Autodesk Fusion 360 part; units mm, degrees
note: some values were not read from the file. Set by a fixed rule: which sketch regions a step uses.
(part 4 of 4)
  spline S327 degree 3 poles (-0.4705, -4.8236) (-0.4586, -4.7125) (-0.5896, -4.4664) (-0.7999, -4.2085) knots 0 0 0 0 1 1 1 1
  line L146 (-0.7999, -4.2085) -> (-0.9586, -4.018)
  line L147 (-0.9586, -4.018) -> (-1.2563, -4.014)
  spline S328 degree 3 poles (-1.2563, -4.014) (-1.4508, -4.014) (-1.6532, -3.9822) (-1.8437, -3.9267) knots 0 0 0 0 1 1 1 1
  spline S329 degree 3 poles (-1.8437, -3.9267) (-2.1771, -3.8235) (-2.1929, -3.8275) (-2.4509, -4.1053) knots 0 0 0 0 1 1 1 1
  spline S330 degree 3 poles (-2.4509, -4.1053) (-2.7366, -4.4109) (-2.7803, -4.4902) (-2.7525, -4.6927) knots 0 0 0 0 1 1 1 1
  spline S331 degree 3 poles (-2.7525, -4.6927) (-2.7208, -4.9189) (-2.5461, -5.3316) (-2.4191, -5.4824) knots 0 0 0 0 1 1 1 1
  spline S332 degree 3 poles (-2.4191, -5.4824) (-2.3041, -5.6213) (-2.3199, -5.6848) (-2.4707, -5.6848) knots 0 0 0 0 1 1 1 1
  spline S333 degree 3 poles (-2.4707, -5.6848) (-2.57, -5.6848) (-2.5977, -5.6571) (-2.6771, -5.4983) knots 0 0 0 0 1 1 1 1
  spline S334 degree 3 poles (-2.6771, -5.4983) (-2.7366, -5.3634) (-2.7882, -5.3078) (-2.8438, -5.3078) knots 0 0 0 0 1 1 1 1
  spline S335 degree 3 poles (-2.8438, -5.3078) (-2.9351, -5.3078) (-2.9351, -5.2959) (-2.9232, -5.792) knots 0 0 0 0 1 1 1 1
  spline S336 degree 3 poles (-2.9232, -5.792) (-2.9192, -6.0023) (-2.9271, -6.1928) (-2.9391, -6.2167) knots 0 0 0 0 1 1 1 1
  spline S337 degree 3 poles (-2.9391, -6.2167) (-2.9589, -6.2444) (-2.9986, -6.2444) (-3.0621, -6.2127) knots 0 0 0 0 1 1 1 1
  spline S338 degree 3 poles (-3.0621, -6.2127) (-3.1772, -6.1611) (-3.2407, -5.9746) (-3.2407, -5.6967) knots 0 0 0 0 1 1 1 1
  spline S339 degree 3 poles (-3.2407, -5.6967) (-3.2407, -5.5896) (-3.2566, -5.5062) (-3.2724, -5.5062) knots 0 0 0 0 1 1 1 1
  spline S340 degree 3 poles (-3.2724, -5.5062) (-3.3359, -5.5062) (-3.4748, -5.6848) (-3.5502, -5.8674) knots 0 0 0 0 1 1 1 1
  spline S341 degree 3 poles (-3.5502, -5.8674) (-3.6455, -6.0897) (-3.7765, -6.1968) (-3.8836, -6.1373) knots 0 0 0 0 1 1 1 1
  spline S342 degree 3 poles (-3.8836, -6.1373) (-3.9789, -6.0857) (-3.9749, -5.9706) (-3.8598, -5.792) knots 0 0 0 0 1 1 1 1
  spline S343 degree 3 poles (-3.8598, -5.792) (-3.7526, -5.6174) (-3.6891, -5.3872) (-3.7526, -5.3872) knots 0 0 0 0 1 1 1 1
  spline S344 degree 3 poles (-3.7526, -5.3872) (-3.7765, -5.3872) (-3.8519, -5.4507) (-3.9233, -5.534) knots 0 0 0 0 1 1 1 1
  spline S345 degree 3 poles (-3.9233, -5.534) (-4.221, -5.8674) (-4.3162, -5.9428) (-4.4353, -5.9428) knots 0 0 0 0 1 1 1 1
  spline S346 degree 3 poles (-4.4353, -5.9428) (-4.6377, -5.9428) (-4.5901, -5.788) (-4.2805, -5.4388) knots 0 0 0 0 1 1 1 1
  spline S347 degree 3 poles (-4.2805, -5.4388) (-4.1297, -5.2681) (-3.9789, -5.1054) (-3.9431, -5.0737) knots 0 0 0 0 1 1 1 1
  spline S348 degree 3 poles (-3.9431, -5.0737) (-3.9035, -5.0459) (-3.8757, -4.9784) (-3.8757, -4.9308) knots 0 0 0 0 1 1 1 1
  spline S349 degree 3 poles (-3.8757, -4.9308) (-3.8757, -4.8435) (-3.8876, -4.8395) (-4.1257, -4.8435) knots 0 0 0 0 1 1 1 1
  spline S350 degree 3 poles (-4.1257, -4.8435) (-4.4075, -4.8514) (-4.4631, -4.78) (-4.2527, -4.6807) knots 0 0 0 0 1 1 1 1
  spline S351 degree 3 poles (-4.2527, -4.6807) (-4.1892, -4.649) (-4.0821, -4.5974) (-4.0225, -4.5696) knots 0 0 0 0 1 1 1 1
  spline S352 degree 3 poles (-4.0225, -4.5696) (-3.959, -4.5379) (-3.84, -4.5141) (-3.7526, -4.5141) knots 0 0 0 0 1 1 1 1
  spline S353 degree 3 poles (-3.7526, -4.5141) (-3.6256, -4.5141) (-3.5621, -4.4823) (-3.3836, -4.3275) knots 0 0 0 0 1 1 1 1
  spline S354 degree 3 poles (-3.3836, -4.3275) (-3.2566, -4.2164) (-3.1653, -4.1013) (-3.1653, -4.0537) knots 0 0 0 0 1 1 1 1
  spline S355 degree 3 poles (-3.1653, -4.0537) (-3.1573, -3.887) (-2.9232, -3.4901) (-2.7366, -3.3393) knots 0 0 0 0 1 1 1 1
  spline S356 degree 3 poles (-2.7366, -3.3393) (-2.5184, -3.1607) (-2.2604, -3.0853) (-1.8675, -3.0853) knots 0 0 0 0 1 1 1 1
  spline S357 degree 3 poles (-1.8675, -3.0853) (-1.6532, -3.0853) (-1.5619, -3.0694) (-1.4984, -3.0178) knots 0 0 0 0 1 1 1 1
  line L148 (-1.4984, -3.0178) -> (-1.4111, -2.9464)
  line L149 (-1.4111, -2.9464) -> (-1.4944, -2.7083)
  spline S358 degree 3 poles (-1.4944, -2.7083) (-1.6413, -2.2955) (-1.7008, -1.9026) (-1.6968, -1.3589) knots 0 0 0 0 1 1 1 1
  spline S359 degree 3 poles (-1.6968, -1.3589) (-1.6968, -0.7477) (-1.5936, -0.2715) (-1.3436, 0.2603) knots 0 0 0 0 1 1 1 1
  line L150 (-1.3436, 0.2603) -> (-1.1888, 0.5937)
  line L151 (-1.1888, 0.5937) -> (-1.3516, 0.558)
  spline S360 degree 3 poles (-1.3516, 0.558) (-1.4389, 0.5342) (-1.6611, 0.5263) (-1.8437, 0.5382) knots 0 0 0 0 1 1 1 1
  spline S361 degree 3 poles (-1.8437, 0.5382) (-2.2644, 0.562) (-2.5858, 0.7048) (-2.6692, 0.9073) knots 0 0 0 0 1 1 1 1
  spline S362 degree 3 poles (-2.6692, 0.9073) (-2.7446, 1.0819) (-2.7406, 1.5462) (-2.6612, 2.0542) knots 0 0 0 0 1 1 1 1
  spline S363 degree 3 poles (-2.6612, 2.0542) (-2.5938, 2.4948) (-2.6017, 2.59) (-2.7128, 2.59) knots 0 0 0 0 1 1 1 1
  spline S364 degree 3 poles (-2.7128, 2.59) (-2.8795, 2.59) (-3.0383, 2.4352) (-3.1811, 2.1376) knots 0 0 0 0 1 1 1 1
  spline S365 degree 3 poles (-3.1811, 2.1376) (-3.328, 1.828) (-3.4193, 1.7407) (-3.5701, 1.7645) knots 0 0 0 0 1 1 1 1
  spline S366 degree 3 poles (-3.5701, 1.7645) (-3.709, 1.7843) (-3.705, 1.955) (-3.5582, 2.0939) knots 0 0 0 0 1 1 1 1
  spline S367 degree 3 poles (-3.5582, 2.0939) (-3.4272, 2.2169) (-3.3994, 2.3519) (-3.5066, 2.3519) knots 0 0 0 0 1 1 1 1
  spline S368 degree 3 poles (-3.5066, 2.3519) (-3.5423, 2.3519) (-3.6852, 2.3082) (-3.8201, 2.2527) knots 0 0 0 0 1 1 1 1
  spline S369 degree 3 poles (-3.8201, 2.2527) (-4.0543, 2.1574) (-4.3638, 2.1138) (-4.4154, 2.1653) knots 0 0 0 0 1 1 1 1
  spline S370 degree 3 poles (-4.4154, 2.1653) (-4.4829, 2.2288) (-4.3757, 2.3519) (-4.221, 2.3916) knots 0 0 0 0 1 1 1 1
  spline S371 degree 3 poles (-4.221, 2.3916) (-3.9947, 2.4471) (-3.6931, 2.6019) (-3.7169, 2.6495) knots 0 0 0 0 1 1 1 1
  spline S372 degree 3 poles (-3.7169, 2.6495) (-3.7288, 2.6694) (-3.7646, 2.6853) (-3.7963, 2.6773) knots 0 0 0 0 1 1 1 1
  spline S373 degree 3 poles (-3.7963, 2.6773) (-4.0582, 2.6218) (-4.3083, 2.594) (-4.6416, 2.594) knots 0 0 0 0 1 1 1 1
  spline S374 degree 3 poles (-4.6416, 2.594) (-5.0187, 2.59) (-5.0306, 2.594) (-5.0187, 2.6773) knots 0 0 0 0 1 1 1 1
  spline S375 degree 3 poles (-5.0187, 2.6773) (-5.0068, 2.7726) (-4.9512, 2.7924) (-4.5305, 2.8678) knots 0 0 0 0 1 1 1 1
  spline S376 degree 3 poles (-4.5305, 2.8678) (-4.1733, 2.9353) (-3.8757, 3.0226) (-3.8757, 3.0623) knots 0 0 0 0 1 1 1 1
  spline S377 degree 3 poles (-3.8757, 3.0623) (-3.8757, 3.1139) (-4.2646, 3.225) (-4.6615, 3.2845) knots 0 0 0 0 1 1 1 1
  spline S378 degree 3 poles (-4.6615, 3.2845) (-5.0742, 3.348) (-5.106, 3.3599) (-5.106, 3.4592) knots 0 0 0 0 1 1 1 1
  spline S379 degree 3 poles (-5.106, 3.4592) (-5.106, 3.6378) (-4.9631, 3.6616) (-4.5385, 3.5385) knots 0 0 0 0 1 1 1 1
  spline S380 degree 3 poles (-4.5385, 3.5385) (-4.3837, 3.4949) (-4.0821, 3.4512) (-3.8757, 3.4393) knots 0 0 0 0 1 1 1 1
  spline S381 degree 3 poles (-3.8757, 3.4393) (-3.5463, 3.4195) (-3.5066, 3.4234) (-3.5701, 3.475) knots 0 0 0 0 1 1 1 1
  spline S382 degree 3 poles (-3.5701, 3.475) (-3.6058, 3.5068) (-3.7288, 3.5425) (-3.84, 3.5544) knots 0 0 0 0 1 1 1 1
  spline S383 degree 3 poles (-3.84, 3.5544) (-4.0741, 3.5822) (-4.1614, 3.6417) (-4.1456, 3.7568) knots 0 0 0 0 1 1 1 1
  spline S384 degree 3 poles (-4.1456, 3.7568) (-4.1336, 3.8322) (-4.1098, 3.8402) (-3.9154, 3.8362) knots 0 0 0 0 1 1 1 1
  spline S385 degree 3 poles (-3.9154, 3.8362) (-3.7963, 3.8322) (-3.5979, 3.7925) (-3.4788, 3.7489) knots 0 0 0 0 1 1 1 1
  spline S386 degree 3 poles (-3.4788, 3.7489) (-2.439, 3.3639) (-2.3596, 3.3282) (-2.1771, 3.1417) knots 0 0 0 0 1 1 1 1
  spline S387 degree 3 poles (-2.1771, 3.1417) (-1.9667, 2.9273) (-1.8119, 2.3955) (-1.8119, 1.8796) knots 0 0 0 0 1 1 1 1
  spline S388 degree 3 poles (-1.8119, 1.8796) (-1.8119, 1.6931) (-1.804, 1.6732) (-1.7445, 1.701) knots 0 0 0 0 1 1 1 1
  spline S389 degree 3 poles (-1.7445, 1.701) (-1.6095, 1.7566) (-1.1571, 1.8717) (-1.0499, 1.8717) knots 0 0 0 0 1 1 1 1
  spline S390 degree 3 poles (-1.0499, 1.8717) (-0.9388, 1.8756) (-0.9388, 1.8756) (-0.9388, 2.1534) knots 0 0 0 0 1 1 1 1
  spline S391 degree 3 poles (-0.9388, 2.1534) (-0.9388, 2.5186) (-0.8356, 2.8202) (-0.5419, 3.3242) knots 0 0 0 0 1 1 1 1
  spline S392 degree 3 poles (-0.5419, 3.3242) (-0.0974, 4.0942) (0.1209, 4.753) (0.1605, 5.4475) knots 0 0 0 0 1 1 1 1
  spline S393 degree 3 poles (0.1605, 5.4475) (0.2161, 6.5389) (-0.2443, 7.1858) (-1.4587, 7.7256) knots 0 0 0 0 1 1 1 1
  spline S394 degree 3 poles (-1.4587, 7.7256) (-1.9786, 7.9558) (-2.9232, 8.0272) (-3.6098, 7.8843) knots 0 0 0 0 1 1 1 1
  spline S395 degree 3 poles (-3.6098, 7.8843) (-4.7647, 7.6502) (-5.6894, 7.0747) (-6.5308, 6.0627) knots 0 0 0 0 1 1 1 1
  line L152 (-6.5308, 6.0627) -> (-6.6617, 5.9039)
  line L153 (-6.6617, 5.9039) -> (-6.5586, 6.1023)
  spline S396 degree 3 poles (-6.5586, 6.1023) (-6.0823, 7.0033) (-5.1298, 7.7414) (-3.9154, 8.1502) knots 0 0 0 0 1 1 1 1
  spline S397 degree 3 poles (-3.9154, 8.1502) (-2.5779, 8.5987) (-1.3595, 8.5908) (-0.2601, 8.1264) knots 0 0 0 0 1 1 1 1
  spline S398 degree 3 poles (-0.2601, 8.1264) (1.5893, 7.3485) (2.006, 6.1063) (1.1884, 3.8322) knots 0 0 0 0 1 1 1 1
  spline S399 degree 3 poles (1.1884, 3.8322) (1.0059, 3.3282) (0.9662, 2.9194) (1.0575, 2.4511) knots 0 0 0 0 1 1 1 1
  spline S400 degree 3 poles (1.0575, 2.4511) (1.1408, 2.0066) (1.1845, 1.9193) (1.3313, 1.8558) knots 0 0 0 0 1 1 1 1
  spline S401 degree 3 poles (1.3313, 1.8558) (1.4028, 1.828) (1.5417, 1.7407) (1.6409, 1.6653) knots 0 0 0 0 1 1 1 1
  line L154 (1.6409, 1.6653) -> (1.8195, 1.5304)
  line L155 (1.8195, 1.5304) -> (1.8195, 1.9709)
  spline S402 degree 3 poles (1.8195, 1.9709) (1.8195, 2.3876) (1.8274, 2.4273) (1.9465, 2.6694) knots 0 0 0 0 1 1 1 1
  spline S403 degree 3 poles (1.9465, 2.6694) (2.1171, 3.0186) (2.2322, 3.1179) (2.7164, 3.3282) knots 0 0 0 0 1 1 1 1
  spline S404 degree 3 poles (2.7164, 3.3282) (3.7165, 3.7687) (4.0658, 3.86) (4.1809, 3.7171) knots 0 0 0 0 1 1 1 1
  spline S405 degree 3 poles (4.1809, 3.7171) (4.2563, 3.6338) (4.1729, 3.5663) (3.9229, 3.5068) knots 0 0 0 0 1 1 1 1
  spline S406 degree 3 poles (3.9229, 3.5068) (3.8118, 3.479) (3.6649, 3.4195) (3.5935, 3.3758) knots 0 0 0 0 1 1 1 1
  spline S407 degree 3 poles (3.5935, 3.3758) (3.4824, 3.3084) (3.4705, 3.2885) (3.5141, 3.2369) knots 0 0 0 0 1 1 1 1
  spline S408 degree 3 poles (3.5141, 3.2369) (3.5538, 3.1853) (3.6292, 3.1814) (3.9428, 3.2012) knots 0 0 0 0 1 1 1 1
  spline S409 degree 3 poles (3.9428, 3.2012) (4.9191, 3.2687) (5.0778, 3.2726) (5.181, 3.229) knots 0 0 0 0 1 1 1 1
  spline S410 degree 3 poles (5.181, 3.229) (5.2961, 3.1853) (5.3318, 3.0782) (5.2405, 3.0464) knots 0 0 0 0 1 1 1 1
  spline S411 degree 3 poles (5.2405, 3.0464) (5.2167, 3.0385) (4.9508, 3.0107) (4.6571, 2.9909) knots 0 0 0 0 1 1 1 1
  spline S412 degree 3 poles (4.6571, 2.9909) (4.0459, 2.9472) (3.8237, 2.8916) (3.911, 2.8004) knots 0 0 0 0 1 1 1 1
  spline S413 degree 3 poles (3.911, 2.8004) (3.9428, 2.7726) (4.038, 2.7369) (4.1253, 2.7249) knots 0 0 0 0 1 1 1 1
  spline S414 degree 3 poles (4.1253, 2.7249) (4.3595, 2.6892) (5.0024, 2.4749) (5.054, 2.4114) knots 0 0 0 0 1 1 1 1
  spline S415 degree 3 poles (5.054, 2.4114) (5.0818, 2.3797) (5.0897, 2.3241) (5.0778, 2.2884) knots 0 0 0 0 1 1 1 1
  spline S416 degree 3 poles (5.0778, 2.2884) (5.0461, 2.209) (4.8635, 2.2289) (4.2999, 2.3757) knots 0 0 0 0 1 1 1 1
  spline S417 degree 3 poles (4.2999, 2.3757) (3.8713, 2.4829) (3.784, 2.4908) (3.784, 2.4194) knots 0 0 0 0 1 1 1 1
  spline S418 degree 3 poles (3.784, 2.4194) (3.784, 2.3519) (3.9269, 2.2169) (4.169, 2.0582) knots 0 0 0 0 1 1 1 1
  spline S419 degree 3 poles (4.169, 2.0582) (4.3595, 1.9352) (4.423, 1.824) (4.3476, 1.7486) knots 0 0 0 0 1 1 1 1
  spline S420 degree 3 poles (4.3476, 1.7486) (4.2761, 1.6772) (4.0737, 1.7566) (3.7999, 1.959) knots 0 0 0 0 1 1 1 1
  spline S421 degree 3 poles (3.7999, 1.959) (3.653, 2.0661) (3.5181, 2.1534) (3.5022, 2.1534) knots 0 0 0 0 1 1 1 1
  spline S422 degree 3 poles (3.5022, 2.1534) (3.4427, 2.1534) (3.4625, 1.9987) (3.5459, 1.8359) knots 0 0 0 0 1 1 1 1
  spline S423 degree 3 poles (3.5459, 1.8359) (3.6491, 1.6335) (3.6491, 1.4549) (3.5499, 1.4272) knots 0 0 0 0 1 1 1 1
  spline S424 degree 3 poles (3.5499, 1.4272) (3.4427, 1.3994) (3.3078, 1.5026) (3.3078, 1.6097) knots 0 0 0 0 1 1 1 1
  spline S425 degree 3 poles (3.3078, 1.6097) (3.3078, 1.7685) (2.9585, 2.209) (2.7839, 2.2685) knots 0 0 0 0 1 1 1 1
  spline S426 degree 3 poles (2.7839, 2.2685) (2.6609, 2.3122) (2.5537, 2.2884) (2.5537, 2.2169) knots 0 0 0 0 1 1 1 1
  spline S427 degree 3 poles (2.5537, 2.2169) (2.5537, 2.1931) (2.5894, 2.0384) (2.6331, 1.8756) knots 0 0 0 0 1 1 1 1
  spline S428 degree 3 poles (2.6331, 1.8756) (2.768, 1.3637) (2.7124, 0.8715) (2.4942, 0.6136) knots 0 0 0 0 1 1 1 1
  spline S429 degree 3 poles (2.4942, 0.6136) (2.3672, 0.4628) (2.2441, 0.4389) (1.8592, 0.5104) knots 0 0 0 0 1 1 1 1
  spline S430 degree 3 poles (1.8592, 0.5104) (1.6845, 0.5382) (1.502, 0.5659) (1.4544, 0.5659) knots 0 0 0 0 1 1 1 1
  line L156 (1.4544, 0.5659) -> (1.367, 0.5659)
  line L157 (1.367, 0.5659) -> (1.4901, 0.2365)
  spline S431 degree 3 poles (1.4901, 0.2365) (1.8869, -0.8152) (2.0139, -1.4541) (1.9862, -2.2519) knots 0 0 0 0 1 1 1 1
  spline S432 degree 3 poles (1.9862, -2.2519) (1.9663, -2.748) (1.9187, -3.002) (1.7838, -3.3274) knots 0 0 0 0 1 1 1 1
  spline S433 degree 3 poles (1.7838, -3.3274) (1.7401, -3.4266) (1.9504, -3.4822) (2.3553, -3.4822) knots 0 0 0 0 1 1 1 1
  spline S434 degree 3 poles (2.3553, -3.4822) (2.6688, -3.4822) (2.7124, -3.4941) (2.895, -3.6052) knots 0 0 0 0 1 1 1 1
  spline S435 degree 3 poles (2.895, -3.6052) (3.0022, -3.6727) (3.1411, -3.7759) (3.2046, -3.8354) knots 0 0 0 0 1 1 1 1
  spline S436 degree 3 poles (3.2046, -3.8354) (3.3236, -3.9426) (3.5062, -4.2878) (3.5062, -4.399) knots 0 0 0 0 1 1 1 1
  spline S437 degree 3 poles (3.5062, -4.399) (3.5062, -4.4664) (3.6927, -4.653) (3.8832, -4.776) knots 0 0 0 0 1 1 1 1
  spline S438 degree 3 poles (3.8832, -4.776) (3.9348, -4.8117) (4.0499, -4.8474) (4.1412, -4.8554) knots 0 0 0 0 1 1 1 1
  spline S439 degree 3 poles (4.1412, -4.8554) (4.3634, -4.8752) (4.7048, -5.0538) (4.6889, -5.1411) knots 0 0 0 0 1 1 1 1
  spline S440 degree 3 poles (4.6889, -5.1411) (4.673, -5.2086) (4.5738, -5.2205) (4.3396, -5.1848) knots 0 0 0 0 1 1 1 1
  spline S441 degree 3 poles (4.3396, -5.1848) (4.2642, -5.1729) (4.2364, -5.1887) (4.2285, -5.2483) knots 0 0 0 0 1 1 1 1
  spline S442 degree 3 poles (4.2285, -5.2483) (4.2206, -5.3038) (4.3436, -5.4546) (4.6174, -5.7325) knots 0 0 0 0 1 1 1 1
  spline S443 degree 3 poles (4.6174, -5.7325) (4.8357, -5.9547) (5.0143, -6.1571) (5.0143, -6.1809) knots 0 0 0 0 1 1 1 1
  spline S444 degree 3 poles (5.0143, -6.1809) (5.0143, -6.2484) (4.8278, -6.2722) (4.6809, -6.2206) knots 0 0 0 0 1 1 1 1
  spline S445 degree 3 poles (4.6809, -6.2206) (4.5936, -6.1928) (4.4825, -6.1016) (4.3912, -5.9904) knots 0 0 0 0 1 1 1 1
  spline S446 degree 3 poles (4.3912, -5.9904) (4.3079, -5.8872) (4.2206, -5.792) (4.2007, -5.7761) knots 0 0 0 0 1 1 1 1
  spline S447 degree 3 poles (4.2007, -5.7761) (4.0658, -5.6769) (4.0698, -5.8356) (4.2087, -6.1174) knots 0 0 0 0 1 1 1 1
  spline S448 degree 3 poles (4.2087, -6.1174) (4.3158, -6.3436) (4.3119, -6.4587) (4.1888, -6.4587) knots 0 0 0 0 1 1 1 1
  spline S449 degree 3 poles (4.1888, -6.4587) (4.0856, -6.4587) (3.9666, -6.3159) (3.8475, -6.0539) knots 0 0 0 0 1 1 1 1
  spline S450 degree 3 poles (3.8475, -6.0539) (3.6927, -5.6967) (3.5856, -5.7642) (3.5856, -6.2127) knots 0 0 0 0 1 1 1 1
  spline S451 degree 3 poles (3.5856, -6.2127) (3.5856, -6.3833) (3.5657, -6.4429) (3.4824, -6.5262) knots 0 0 0 0 1 1 1 1
  spline S452 degree 3 poles (3.4824, -6.5262) (3.3911, -6.6175) (3.3752, -6.6215) (3.3197, -6.5699) knots 0 0 0 0 1 1 1 1
  spline S453 degree 3 poles (3.3197, -6.5699) (3.272, -6.5183) (3.2681, -6.4786) (3.3038, -6.3556) knots 0 0 0 0 1 1 1 1
  spline S454 degree 3 poles (3.3038, -6.3556) (3.3594, -6.1571) (3.3594, -5.8396) (3.3078, -5.7404) knots 0 0 0 0 1 1 1 1
  spline S455 degree 3 poles (3.3078, -5.7404) (3.2324, -5.6015) (3.1173, -5.6491) (3.0101, -5.8634) knots 0 0 0 0 1 1 1 1
  spline S456 degree 3 poles (3.0101, -5.8634) (2.9387, -6.0063) (2.8871, -6.0619) (2.8275, -6.0619) knots 0 0 0 0 1 1 1 1
  spline S457 degree 3 poles (2.8275, -6.0619) (2.7283, -6.0619) (2.7402, -6.0182) (2.9387, -5.5697) knots 0 0 0 0 1 1 1 1
  spline S458 degree 3 poles (2.9387, -5.5697) (3.0895, -5.2364) (3.1331, -5.0181) (3.0934, -4.8514) knots 0 0 0 0 1 1 1 1
  spline S459 degree 3 poles (3.0934, -4.8514) (3.0657, -4.7363) (2.8514, -4.4902) (2.6331, -4.3156) knots 0 0 0 0 1 1 1 1
  line L158 (2.6331, -4.3156) -> (2.4862, -4.2005)
  line L159 (2.4862, -4.2005) -> (2.1767, -4.2997)
  spline S460 degree 3 poles (2.1767, -4.2997) (1.9782, -4.3632) (1.7679, -4.399) (1.5853, -4.4029) knots 0 0 0 0 1 1 1 1
  line L160 (1.5853, -4.4029) -> (1.3035, -4.4069)
  line L161 (1.3035, -4.4069) -> (1.1289, -4.6252)
  spline S461 degree 3 poles (1.1289, -4.6252) (0.9305, -4.8752) (0.863, -5.0697) (0.9265, -5.1887) knots 0 0 0 0 1 1 1 1
  spline S462 degree 3 poles (0.9265, -5.1887) (0.9503, -5.2324) (0.9821, -5.2681) (1.0019, -5.2681) knots 0 0 0 0 1 1 1 1
  spline S463 degree 3 poles (1.0019, -5.2681) (1.0773, -5.2681) (1.3234, -5.5697) (1.3789, -5.7364) knots 0 0 0 0 1 1 1 1
  spline S464 degree 3 poles (1.3789, -5.7364) (1.4504, -5.9428) (1.4623, -6.5183) (1.4028, -6.7405) knots 0 0 0 0 1 1 1 1
  spline S465 degree 3 poles (1.4028, -6.7405) (1.3789, -6.8199) (1.3194, -6.9469) (1.2639, -7.0183) knots 0 0 0 0 1 1 1 1
  spline S466 degree 3 poles (1.2639, -7.0183) (1.2123, -7.0937) (1.1408, -7.2128) (1.1091, -7.2803) knots 0 0 0 0 1 1 1 1
  spline S467 degree 3 poles (1.1091, -7.2803) (1.0773, -7.3517) (0.9979, -7.4867) (0.9344, -7.5779) knots 0 0 0 0 1 1 1 1
  spline S468 degree 3 poles (0.9344, -7.5779) (0.8709, -7.6732) (0.7638, -7.8637) (0.7003, -8.0066) knots 0 0 0 0 1 1 1 1
  spline S469 degree 3 poles (0.7003, -8.0066) (0.5733, -8.2883) (0.3788, -8.5304) (0.1923, -8.6495) knots 0 0 0 0 1 1 1 1
  spline S470 degree 3 poles (-7.5547, -14.3566) (-7.5706, -14.3566) (-7.7452, -14.2653) (-7.9436, -14.1502) knots 0 0 0 0 1 1 1 1
  spline S471 degree 3 poles (-7.9436, -14.1502) (-8.8287, -13.6462) (-9.0192, -13.4239) (-8.789, -13.1778) knots 0 0 0 0 1 1 1 1
  spline S472 degree 3 poles (-8.789, -13.1778) (-8.6302, -13.0072) (-8.3881, -13.0707) (-7.6896, -13.4676) knots 0 0 0 0 1 1 1 1
  spline S473 degree 3 poles (-7.6896, -13.4676) (-7.4356, -13.6144) (-7.2213, -13.7414) (-7.2094, -13.7493) knots 0 0 0 0 1 1 1 1
  spline S474 degree 3 poles (-7.2094, -13.7493) (-7.1777, -13.7771) (-7.5031, -14.3566) (-7.5547, -14.3566) knots 0 0 0 0 1 1 1 1
  spline S475 degree 3 poles (-0.1609, 15.1789) (-0.7007, 15.1908) (-0.7801, 15.1987) (-0.8555, 15.2662) knots 0 0 0 0 1 1 1 1
  spline S476 degree 3 poles (-0.8555, 15.2662) (-0.915, 15.3218) (-0.9388, 15.3813) (-0.9309, 15.4646) knots 0 0 0 0 1 1 1 1
  spline S477 degree 3 poles (-0.9309, 15.4646) (-0.911, 15.6591) (-0.7404, 15.7147) (-0.0974, 15.7464) knots 0 0 0 0 1 1 1 1
  line L162 (-0.0974, 15.7464) -> (0.4503, 15.7742)
  line L163 (0.4503, 15.7742) -> (0.4503, 15.167)
  line L164 (0.4503, 15.167) -> (-0.1609, 15.1789)
  spline S478 degree 3 poles (-13.0594, -9.7806) (-13.0792, -9.7727) (-13.2181, -9.5901) (-13.3689, -9.3718) knots 0 0 0 0 1 1 1 1
  spline S479 degree 3 poles (-13.3689, -9.3718) (-13.9682, -8.4987) (-13.9484, -8.0542) (-13.2935, -7.7168) knots 0 0 0 0 1 1 1 1
  spline S480 degree 3 poles (-13.2935, -7.7168) (-13.0117, -7.57) (-12.6506, -7.6772) (-12.3648, -7.9907) knots 0 0 0 0 1 1 1 1
  spline S481 degree 3 poles (-12.3648, -7.9907) (-12.2061, -8.1653) (-11.7298, -8.8479) (-11.7417, -8.8876) knots 0 0 0 0 1 1 1 1
  spline S482 degree 3 poles (-11.7417, -8.8876) (-11.7616, -8.9432) (-13.0157, -9.7965) (-13.0594, -9.7806) knots 0 0 0 0 1 1 1 1
  spline S483 degree 3 poles (-4.729, 14.4645) (-4.8877, 14.4724) (-5.0068, 14.5042) (-5.0742, 14.5558) knots 0 0 0 0 1 1 1 1
  spline S484 degree 3 poles (-5.0742, 14.5558) (-5.3441, 14.7582) (-5.4354, 15.1908) (-5.2687, 15.4646) knots 0 0 0 0 1 1 1 1
  spline S485 degree 3 poles (-5.2687, 15.4646) (-5.0782, 15.7742) (-4.4829, 15.9131) (-4.1892, 15.7147) knots 0 0 0 0 1 1 1 1
  spline S486 degree 3 poles (-4.1892, 15.7147) (-4.0265, 15.6075) (-3.8757, 15.3257) (-3.8757, 15.1313) knots 0 0 0 0 1 1 1 1
  spline S487 degree 3 poles (-3.8757, 15.1313) (-3.8796, 14.7503) (-4.2765, 14.4367) (-4.729, 14.4645) knots 0 0 0 0 1 1 1 1
extrude "Extrude7''" cut sketch "Sketch4" against normal blind 1 contours S0 S1 S2 L4 L5 S3 | S49 S50 S51 S52 S53 S54 S55 | S56 S57 S58 S59 | S60 S61 S62 S63 | S64 S65 S66 S67 S68 | S69 S70 S71 S72 | S148 S149 S150 S151 | S152 S153 S154 S155 S156 | S157 S158 S159 S160 | S306 S307 S308 S309 S310 S311 S312 S313 S314 S315 S316 S317 S318 | S319 S320 S321 S322 S323 S324 S325 S326 S327 L146 L147 S328 S329 S330 S331 S332 S333 S334 S335 S336 S337 S338 S339 S340 S341 S342 S343 S344 S345 S346 S347 S348 S349 S350 S351 S352 S353 S354 S355 S356 S357 L148 L149 S358 S359 L150 L151 S360 S361 S362 S363 S364 S365 S366 S367 S368 S369 S370 S371 S372 S373 S374 S375 S376 S377 S378 S379 S380 S381 S382 S383 S384 S385 S386 S387 S388 S389 S390 S391 S392 S393 S394 S395 L152 L153 S396 S397 S398 S399 S400 S401 L154 L155 S402 S403 S404 S405 S406 S407 S408 S409 S410 S411 S412 S413 S414 S415 S416 S417 S418 S419 S420 S421 S422 S423 S424 S425 S426 S427 S428 S429 S430 L156 L157 S431 S432 S433 S434 S435 S436 S437 S438 S439 S440 S441 S442 S443 S444 S445 S446 S447 S448 S449 S450 S451 S452 S453 S454 S455 S456 S457 S458 S459 L158 L159 S460 L160 L161 S461 S462 S463 S464 S465 S466 S467 S468 S469 | S470 S471 S472 S473 S474 | S475 S476 S477 L162 L163 L164 | S478 S479 S480 S481 S482 | S483 S484 S485 S486 S487 bodies 3 in component "Enclosure_Bottom"
component "PCB" placed x (1, 0, 0) y (0, 1, 0) z (0, 0, 1) at (0, 0, 7.5)
component "Enclosure_Top" placed x (1, 0, 0) y (0, 1, 0) z (0, 0, 1) at (0, 0, 0)
component "Enclosure_Bottom" placed x (1, 0, 0) y (0, 1, 0) z (0, 0, 1) at (0, 0, 0)
component "_Logo v2" placed x (-1, 0, 0) y (0, 0, -1) z (0, -1, 0) at (145.5531, 138.9899, 0)
